Autodesk Inventor part; units mm, degrees
(part 2 of 3)
  line L370 (-43.7992, -26.7716) -> (-40.2132, -24.3987)
  spline S220 degree 2 poles (-43.3093, -22.1277) (-42.5945, -21.7354) (-41.4383, -21.9952) (-41.1231, -22.5695) knots 0 0 0 1 2 2 2
  spline S221 degree 2 poles (-41.1231, -22.5695) (-40.7995, -23.159) (-41.2324, -24.2751) (-41.9227, -24.654) knots 0 0 0 1 2 2 2
  spline S222 degree 2 poles (-41.9227, -24.654) (-42.6314, -25.043) (-43.7988, -24.7774) (-44.1106, -24.2092) knots 0 0 0 1 2 2 2
  spline S223 degree 2 poles (-44.1106, -24.2092) (-44.4258, -23.6349) (-44.0211, -22.5184) (-43.3093, -22.1277) knots 0 0 0 1 2 2 2
  spline S224 degree 2 poles (-43.0394, -22.6196) (-43.5892, -22.9214) (-43.9042, -23.6149) (-43.7013, -23.9846) knots 0 0 0 1 2 2 2
  spline S225 degree 2 poles (-43.7013, -23.9846) (-43.4984, -24.3542) (-42.7425, -24.464) (-42.1927, -24.1622) knots 0 0 0 1 2 2 2
  spline S226 degree 2 poles (-42.1927, -24.1622) (-41.6581, -23.8688) (-41.3296, -23.1638) (-41.5325, -22.7941) knots 0 0 0 1 2 2 2
  spline S227 degree 2 poles (-41.5325, -22.7941) (-41.7337, -22.4276) (-42.4957, -22.3211) (-43.0394, -22.6196) knots 0 0 0 1 2 2 2
  line L371 (-45.2535, -20.4403) -> (-45.2415, -20.4655)
  spline S228 degree 2 poles (-45.2415, -20.4655) (-45.2302, -20.5296) (-45.178, -20.6552) (-45.1375, -20.7401) knots 0 0 0 1 2 2 2
  spline S229 degree 2 poles (-45.1375, -20.7401) (-45.0429, -20.9383) (-44.6839, -21.2457) (-44.4301, -21.3408) knots 0 0 0 1 2 2 2
  line L372 (-44.4301, -21.3408) -> (-42.3638, -20.355)
  line L373 (-42.3638, -20.355) -> (-42.1297, -20.8456)
  line L374 (-42.1297, -20.8456) -> (-45.042, -22.2351)
  line L375 (-45.042, -22.2351) -> (-45.2761, -21.7445)
  line L376 (-45.2761, -21.7445) -> (-44.842, -21.5374)
  spline S230 degree 2 poles (-44.842, -21.5374) (-45.2086, -21.3841) (-45.5942, -21.0777) (-45.6842, -20.889) knots 0 0 0 1 2 2 2
  spline S231 degree 2 poles (-45.6842, -20.889) (-45.7202, -20.8135) (-45.7499, -20.7351) (-45.763, -20.6834) knots 0 0 0 1 2 2 2
  line L377 (-45.763, -20.6834) -> (-45.2535, -20.4403)
  spline S232 degree 2 poles (-45.6388, -17.058) (-44.8904, -16.7524) (-43.7153, -17.1043) (-43.4927, -17.6495) knots 0 0 0 1 2 2 2
  spline S233 degree 2 poles (-43.4927, -17.6495) (-43.4018, -17.8721) (-43.3654, -18.2562) (-43.3994, -18.4771) knots 0 0 0 1 2 2 2
  line L378 (-43.3994, -18.4771) -> (-42.1477, -17.9659)
  line L379 (-42.1477, -17.9659) -> (-41.9422, -18.4692)
  line L380 (-41.9422, -18.4692) -> (-46.0294, -20.1384)
  line L381 (-46.0294, -20.1384) -> (-46.235, -19.6351)
  line L382 (-46.235, -19.6351) -> (-45.9221, -19.5074)
  spline S234 degree 2 poles (-45.9221, -19.5074) (-46.1694, -19.3901) (-46.5823, -19.0242) (-46.6917, -18.7565) knots 0 0 0 1 2 2 2
  spline S235 degree 2 poles (-46.6917, -18.7565) (-46.9012, -18.2435) (-46.3227, -17.3373) (-45.6388, -17.058) knots 0 0 0 1 2 2 2
  spline S236 degree 2 poles (-45.3687, -17.5537) (-45.8816, -17.7631) (-46.3131, -18.3195) (-46.1642, -18.6841) knots 0 0 0 1 2 2 2
  spline S237 degree 2 poles (-46.1642, -18.6841) (-46.0772, -18.897) (-45.7235, -19.2193) (-45.5027, -19.3361) knots 0 0 0 1 2 2 2
  line L383 (-45.5027, -19.3361) -> (-43.8058, -18.6431)
  spline S238 degree 2 poles (-43.8058, -18.6431) (-43.7926, -18.4081) (-43.8363, -18.0985) (-43.9101, -17.9178) knots 0 0 0 1 2 2 2
  spline S239 degree 2 poles (-43.9101, -17.9178) (-44.0695, -17.5275) (-44.8202, -17.3297) (-45.3687, -17.5537) knots 0 0 0 1 2 2 2
  line L384 (-45.0446, -13.4768) -> (-44.8746, -13.9931)
  line L385 (-44.8746, -13.9931) -> (-46.6223, -14.5683)
  spline S240 degree 2 poles (-46.6223, -14.5683) (-46.8341, -14.638) (-47.1852, -14.7975) (-47.2748, -14.893) knots 0 0 0 1 2 2 2
  spline S241 degree 2 poles (-47.2748, -14.893) (-47.3699, -14.994) (-47.4084, -15.2562) (-47.3452, -15.4481) knots 0 0 0 1 2 2 2
  spline S242 degree 2 poles (-47.3452, -15.4481) (-47.2821, -15.6401) (-46.9429, -15.9797) (-46.7131, -16.1205) knots 0 0 0 1 2 2 2
  line L386 (-46.7131, -16.1205) -> (-44.4226, -15.3668)
  line L387 (-44.4226, -15.3668) -> (-44.2527, -15.8831)
  line L388 (-44.2527, -15.8831) -> (-48.5192, -17.2872)
  line L389 (-48.5192, -17.2872) -> (-48.6892, -16.7708)
  line L390 (-48.6892, -16.7708) -> (-47.1467, -16.2632)
  spline S243 degree 2 poles (-47.1467, -16.2632) (-47.4315, -16.1002) (-47.797, -15.7252) (-47.8798, -15.4736) knots 0 0 0 1 2 2 2
  spline S244 degree 2 poles (-47.8798, -15.4736) (-48.0279, -15.0235) (-47.5999, -14.3177) (-47.0339, -14.1314) knots 0 0 0 1 2 2 2
  line L391 (-47.0339, -14.1314) -> (-45.0446, -13.4768)
  spline S245 degree 2 poles (-47.472, -10.5709) (-46.6817, -10.3701) (-45.6275, -10.9113) (-45.4662, -11.5462) knots 0 0 0 1 2 2 2
  spline S246 degree 2 poles (-45.4662, -11.5462) (-45.3006, -12.1981) (-45.9993, -13.1701) (-46.7626, -13.3639) knots 0 0 0 1 2 2 2
  spline S247 degree 2 poles (-46.7626, -13.3639) (-47.5462, -13.563) (-48.6097, -13.0134) (-48.7693, -12.3852) knots 0 0 0 1 2 2 2
  spline S248 degree 2 poles (-48.7693, -12.3852) (-48.9305, -11.7502) (-48.2589, -10.7707) (-47.472, -10.5709) knots 0 0 0 1 2 2 2
  spline S249 degree 2 poles (-47.3339, -11.1146) (-47.9418, -11.269) (-48.4205, -11.8616) (-48.3167, -12.2702) knots 0 0 0 1 2 2 2
  spline S250 degree 2 poles (-48.3167, -12.2702) (-48.2129, -12.6789) (-47.5086, -12.9746) (-46.9007, -12.8202) knots 0 0 0 1 2 2 2
  spline S251 degree 2 poles (-46.9007, -12.8202) (-46.3097, -12.6701) (-45.815, -12.0698) (-45.9188, -11.6612) knots 0 0 0 1 2 2 2
  spline S252 degree 2 poles (-45.9188, -11.6612) (-46.0217, -11.2559) (-46.7327, -10.9619) (-47.3339, -11.1146) knots 0 0 0 1 2 2 2
  spline S253 degree 2 poles (-49.7235, -5.5011) (-49.4475, -5.4621) (-48.9228, -5.5884) (-48.7254, -5.7399) knots 0 0 0 1 2 2 2
  spline S254 degree 2 poles (-48.7254, -5.7399) (-48.4768, -5.93) (-48.168, -6.4951) (-48.1036, -6.9505) knots 0 0 0 1 2 2 2
  line L392 (-48.1036, -6.9505) -> (-48.0357, -7.4301)
  line L393 (-48.0357, -7.4301) -> (-46.4486, -7.2054)
  line L394 (-46.4486, -7.2054) -> (-46.3685, -7.7713)
  line L395 (-46.3685, -7.7713) -> (-50.626, -8.374)
  line L396 (-50.626, -8.374) -> (-50.7774, -7.3044)
  spline S255 degree 2 poles (-50.7774, -7.3044) (-50.8312, -6.9249) (-50.7822, -6.376) (-50.6695, -6.1524) knots 0 0 0 1 2 2 2
  spline S256 degree 2 poles (-50.6695, -6.1524) (-50.5411, -5.8914) (-50.0789, -5.5515) (-49.7235, -5.5011) knots 0 0 0 1 2 2 2
  spline S257 degree 2 poles (-49.6228, -6.0887) (-49.8436, -6.1199) (-50.1464, -6.3177) (-50.2279, -6.4876) knots 0 0 0 1 2 2 2
  spline S258 degree 2 poles (-50.2279, -6.4876) (-50.2986, -6.6348) (-50.3202, -7.0039) (-50.2826, -7.2696) knots 0 0 0 1 2 2 2
  line L397 (-50.2826, -7.2696) -> (-50.2162, -7.7388)
  line L398 (-50.2162, -7.7388) -> (-48.5187, -7.4985)
  line L399 (-48.5187, -7.4985) -> (-48.5734, -7.1121)
  spline S259 degree 2 poles (-48.5734, -7.1121) (-48.6222, -6.7671) (-48.7927, -6.3583) (-48.9572, -6.2408) knots 0 0 0 1 2 2 2
  spline S260 degree 2 poles (-48.9572, -6.2408) (-49.1029, -6.1312) (-49.4192, -6.0599) (-49.6228, -6.0887) knots 0 0 0 1 2 2 2
  line L400 (-46.9725, -2.0535) -> (-46.934, -2.5957)
  line L401 (-46.934, -2.5957) -> (-48.7693, -2.7261)
  spline S261 degree 2 poles (-48.7693, -2.7261) (-48.9917, -2.7419) (-49.3711, -2.8107) (-49.4814, -2.8814) knots 0 0 0 1 2 2 2
  spline S262 degree 2 poles (-49.4814, -2.8814) (-49.5983, -2.9561) (-49.6997, -3.2009) (-49.6854, -3.4025) knots 0 0 0 1 2 2 2
  spline S263 degree 2 poles (-49.6854, -3.4025) (-49.6711, -3.6041) (-49.4252, -4.0163) (-49.2369, -4.209) knots 0 0 0 1 2 2 2
  line L402 (-49.2369, -4.209) -> (-46.8316, -4.0382)
  line L403 (-46.8316, -4.0382) -> (-46.7931, -4.5805)
  line L404 (-46.7931, -4.5805) -> (-51.2735, -4.8986)
  line L405 (-51.2735, -4.8986) -> (-51.312, -4.3564)
  line L406 (-51.312, -4.3564) -> (-49.6922, -4.2414)
  spline S264 degree 2 poles (-49.6922, -4.2414) (-49.9285, -4.0136) (-50.1912, -3.5607) (-50.21, -3.2965) knots 0 0 0 1 2 2 2
  spline S265 degree 2 poles (-50.21, -3.2965) (-50.2435, -2.8238) (-49.6559, -2.2441) (-49.0615, -2.2019) knots 0 0 0 1 2 2 2
  line L407 (-49.0615, -2.2019) -> (-46.9725, -2.0535)
  line L408 (-50.2328, 1.2276) -> (-45.81, -0.4878)
  line L409 (-45.81, -0.4878) -> (-45.8074, -1.0697)
  line L410 (-45.8074, -1.0697) -> (-47.155, -0.4973)
  line L411 (-47.155, -0.4973) -> (-50.2196, -1.682)
  line L412 (-50.2196, -1.682) -> (-50.2223, -1.0966)
  line L413 (-50.2223, -1.0966) -> (-47.8359, -0.2042)
  line L414 (-47.8359, -0.2042) -> (-50.2303, 0.6631)
  line L415 (-50.2303, 0.6631) -> (-50.2328, 1.2276)
  spline S266 degree 2 poles (-46.8557, 2.5183) (-46.8735, 2.1947) (-47.0782, 1.6441) (-47.1858, 1.465) knots 0 0 0 1 2 2 2
  line L416 (-47.1858, 1.465) -> (-47.7947, 1.4984)
  line L417 (-47.7947, 1.4984) -> (-47.7931, 1.5263)
  spline S267 degree 2 poles (-47.7931, 1.5263) (-47.7336, 1.5928) (-47.5911, 1.7734) (-47.5095, 1.926) knots 0 0 0 1 2 2 2
  spline S268 degree 2 poles (-47.5095, 1.926) (-47.4359, 2.0581) (-47.3201, 2.3867) (-47.3104, 2.5642) knots 0 0 0 1 2 2 2
  spline S269 degree 2 poles (-47.3104, 2.5642) (-47.3033, 2.6929) (-47.3462, 2.9919) (-47.3911, 3.0642) knots 0 0 0 1 2 2 2
  spline S270 degree 2 poles (-47.3911, 3.0642) (-47.4517, 3.1687) (-47.5963, 3.2674) (-47.7494, 3.2758) knots 0 0 0 1 2 2 2
  spline S271 degree 2 poles (-47.7494, 3.2758) (-47.9408, 3.2863) (-48.1506, 3.0884) (-48.2314, 2.8241) knots 0 0 0 1 2 2 2
  spline S272 degree 2 poles (-48.2314, 2.8241) (-48.2615, 2.7211) (-48.3494, 2.3909) (-48.3955, 2.2503) knots 0 0 0 1 2 2 2
  spline S273 degree 2 poles (-48.3955, 2.2503) (-48.5236, 1.8874) (-48.9873, 1.5779) (-49.3039, 1.5953) knots 0 0 0 1 2 2 2
  spline S274 degree 2 poles (-49.3039, 1.5953) (-49.7423, 1.6193) (-50.2525, 2.3069) (-50.2227, 2.8497) knots 0 0 0 1 2 2 2
  spline S275 degree 2 poles (-50.2227, 2.8497) (-50.208, 3.1176) (-50.046, 3.6531) (-49.935, 3.832) knots 0 0 0 1 2 2 2
  line L418 (-49.935, 3.832) -> (-49.3539, 3.8001)
  line L419 (-49.3539, 3.8001) -> (-49.3554, 3.7723)
  spline S276 degree 2 poles (-49.3554, 3.7723) (-49.5339, 3.5727) (-49.7532, 3.0752) (-49.7675, 2.8142) knots 0 0 0 1 2 2 2
  spline S277 degree 2 poles (-49.7675, 2.8142) (-49.7822, 2.5463) (-49.5763, 2.1651) (-49.3501, 2.1527) knots 0 0 0 1 2 2 2
  spline S278 degree 2 poles (-49.3501, 2.1527) (-49.1448, 2.1414) (-48.9345, 2.3497) (-48.8585, 2.5898) knots 0 0 0 1 2 2 2
  spline S279 degree 2 poles (-48.8585, 2.5898) (-48.8207, 2.7064) (-48.7416, 3.0022) (-48.6944, 3.1636) knots 0 0 0 1 2 2 2
  spline S280 degree 2 poles (-48.6944, 3.1636) (-48.5844, 3.5136) (-48.1505, 3.8527) (-47.7921, 3.833) knots 0 0 0 1 2 2 2
  spline S281 degree 2 poles (-47.7921, 3.833) (-47.5834, 3.8216) (-47.2235, 3.6378) (-47.0966, 3.4703) knots 0 0 0 1 2 2 2
  spline S282 degree 2 poles (-47.0966, 3.4703) (-46.9633, 3.292) (-46.8376, 2.8488) (-46.8557, 2.5183) knots 0 0 0 1 2 2 2
  line L420 (-46.7514, 4.8356) -> (-46.8042, 4.2945)
  line L421 (-46.8042, 4.2945) -> (-50.0157, 4.6079)
  line L422 (-50.0157, 4.6079) -> (-49.9629, 5.149)
  line L423 (-49.9629, 5.149) -> (-46.7514, 4.8356)
  line L424 (-50.4932, 5.2392) -> (-50.5531, 4.6254)
  line L425 (-50.5531, 4.6254) -> (-51.115, 4.6802)
  line L426 (-51.115, 4.6802) -> (-51.0551, 5.2941)
  line L427 (-51.0551, 5.2941) -> (-50.4932, 5.2392)
  spline S283 degree 2 poles (-46.4195, 6.8888) (-46.4664, 6.5576) (-46.7476, 6.0378) (-46.9825, 5.8705) knots 0 0 0 1 2 2 2
  spline S284 degree 2 poles (-46.9825, 5.8705) (-47.2139, 5.7027) (-47.8726, 5.5742) (-48.2935, 5.6338) knots 0 0 0 1 2 2 2
  spline S285 degree 2 poles (-48.2935, 5.6338) (-48.7145, 5.6934) (-49.2968, 6.0047) (-49.477, 6.2237) knots 0 0 0 1 2 2 2
  spline S286 degree 2 poles (-49.477, 6.2237) (-49.6606, 6.4433) (-49.8052, 7.0374) (-49.7593, 7.3618) knots 0 0 0 1 2 2 2
  spline S287 degree 2 poles (-49.7593, 7.3618) (-49.7221, 7.624) (-49.5044, 8.0929) (-49.3809, 8.269) knots 0 0 0 1 2 2 2
  line L428 (-49.3809, 8.269) -> (-48.7771, 8.1835)
  line L429 (-48.7771, 8.1835) -> (-48.7815, 8.1524)
  spline S288 degree 2 poles (-48.7815, 8.1524) (-48.8381, 8.1006) (-48.9877, 7.9388) (-49.0714, 7.8204) knots 0 0 0 1 2 2 2
  spline S289 degree 2 poles (-49.0714, 7.8204) (-49.1427, 7.7144) (-49.272, 7.423) (-49.2915, 7.285) knots 0 0 0 1 2 2 2
  spline S290 degree 2 poles (-49.2915, 7.285) (-49.3506, 6.8675) (-48.7911, 6.2709) (-48.2149, 6.1893) knots 0 0 0 1 2 2 2
  spline S291 degree 2 poles (-48.2149, 6.1893) (-47.6525, 6.1097) (-46.9517, 6.5102) (-46.8902, 6.9449) knots 0 0 0 1 2 2 2
  spline S292 degree 2 poles (-46.8902, 6.9449) (-46.853, 7.2071) (-47.003, 7.714) (-47.1461, 7.9208) knots 0 0 0 1 2 2 2
  line L430 (-47.1461, 7.9208) -> (-47.1417, 7.9519)
  line L431 (-47.1417, 7.9519) -> (-46.538, 7.8664)
  spline S293 degree 2 poles (-46.538, 7.8664) (-46.5112, 7.7816) (-46.4385, 7.525) (-46.428, 7.4249) knots 0 0 0 1 2 2 2
  spline S294 degree 2 poles (-46.428, 7.4249) (-46.4062, 7.2811) (-46.3955, 7.0579) (-46.4195, 6.8888) knots 0 0 0 1 2 2 2
  spline S295 degree 2 poles (-46.0194, 9.166) (-46.0831, 8.8482) (-46.3641, 8.3324) (-46.4961, 8.1705) knots 0 0 0 1 2 2 2
  line L432 (-46.4961, 8.1705) -> (-47.094, 8.2903)
  line L433 (-47.094, 8.2903) -> (-47.0885, 8.3176)
  spline S296 degree 2 poles (-47.0885, 8.3176) (-47.0202, 8.375) (-46.8534, 8.5335) (-46.7508, 8.6728) knots 0 0 0 1 2 2 2
  spline S297 degree 2 poles (-46.7508, 8.6728) (-46.6592, 8.7931) (-46.4978, 9.1019) (-46.4629, 9.2762) knots 0 0 0 1 2 2 2
  spline S298 degree 2 poles (-46.4629, 9.2762) (-46.4376, 9.4026) (-46.4375, 9.7046) (-46.4716, 9.7826) knots 0 0 0 1 2 2 2
  spline S299 degree 2 poles (-46.4716, 9.7826) (-46.5167, 9.8947) (-46.6458, 10.0129) (-46.7961, 10.0431) knots 0 0 0 1 2 2 2
  spline S300 degree 2 poles (-46.7961, 10.0431) (-46.984, 10.0807) (-47.2199, 9.9147) (-47.3375, 9.6646) knots 0 0 0 1 2 2 2
  spline S301 degree 2 poles (-47.3375, 9.6646) (-47.382, 9.5669) (-47.516, 9.2526) (-47.5817, 9.1201) knots 0 0 0 1 2 2 2
  spline S302 degree 2 poles (-47.5817, 9.1201) (-47.7601, 8.7791) (-48.2632, 8.5388) (-48.5741, 8.6011) knots 0 0 0 1 2 2 2
  spline S303 degree 2 poles (-48.5741, 8.6011) (-49.0046, 8.6873) (-49.4117, 9.4406) (-49.3049, 9.9736) knots 0 0 0 1 2 2 2
  spline S304 degree 2 poles (-49.3049, 9.9736) (-49.2521, 10.2366) (-49.0155, 10.7436) (-48.8801, 10.9049) knots 0 0 0 1 2 2 2
  line L434 (-48.8801, 10.9049) -> (-48.3096, 10.7905)
  line L435 (-48.3096, 10.7905) -> (-48.315, 10.7632)
  spline S305 degree 2 poles (-48.315, 10.7632) (-48.5201, 10.5911) (-48.808, 10.1299) (-48.8593, 9.8736) knots 0 0 0 1 2 2 2
  spline S306 degree 2 poles (-48.8593, 9.8736) (-48.912, 9.6105) (-48.7625, 9.2039) (-48.5404, 9.1594) knots 0 0 0 1 2 2 2
  spline S307 degree 2 poles (-48.5404, 9.1594) (-48.3389, 9.119) (-48.101, 9.2952) (-47.9916, 9.5221) knots 0 0 0 1 2 2 2
  spline S308 degree 2 poles (-47.9916, 9.5221) (-47.9375, 9.6321) (-47.8171, 9.9136) (-47.7474, 10.0666) knots 0 0 0 1 2 2 2
  spline S309 degree 2 poles (-47.7474, 10.0666) (-47.5887, 10.3973) (-47.1109, 10.6712) (-46.759, 10.6007) knots 0 0 0 1 2 2 2
  spline S310 degree 2 poles (-46.759, 10.6007) (-46.554, 10.5596) (-46.224, 10.3265) (-46.1223, 10.1426) knots 0 0 0 1 2 2 2
  spline S311 degree 2 poles (-46.1223, 10.1426) (-46.0157, 9.9471) (-45.9544, 9.4906) (-46.0194, 9.166) knots 0 0 0 1 2 2 2
  line L436 (-45.1171, 18.2845) -> (-45.6167, 16.9164)
  line L437 (-45.6167, 16.9164) -> (-44.2485, 16.4167)
  line L438 (-44.2485, 16.4167) -> (-44.4135, 15.965)
  line L439 (-44.4135, 15.965) -> (-45.7817, 16.4647)
  line L440 (-45.7817, 16.4647) -> (-46.2813, 15.0965)
  line L441 (-46.2813, 15.0965) -> (-46.7166, 15.2554)
  line L442 (-46.7166, 15.2554) -> (-46.217, 16.6236)
  line L443 (-46.217, 16.6236) -> (-47.5852, 17.1233)
  line L444 (-47.5852, 17.1233) -> (-47.4202, 17.575)
  line L445 (-47.4202, 17.575) -> (-46.052, 17.0753)
  line L446 (-46.052, 17.0753) -> (-45.5524, 18.4435)
  line L447 (-45.5524, 18.4435) -> (-45.1171, 18.2845)
  line L448 (-43.2576, 22.3305) -> (-43.8802, 21.0137)
  line L449 (-43.8802, 21.0137) -> (-42.5634, 20.3911)
  line L450 (-42.5634, 20.3911) -> (-42.7689, 19.9564)
  line L451 (-42.7689, 19.9564) -> (-44.0857, 20.5789)
  line L452 (-44.0857, 20.5789) -> (-44.7083, 19.2621)
  line L453 (-44.7083, 19.2621) -> (-45.1273, 19.4602)
  line L454 (-45.1273, 19.4602) -> (-44.5047, 20.777)
  line L455 (-44.5047, 20.777) -> (-45.8215, 21.3996)
  line L456 (-45.8215, 21.3996) -> (-45.616, 21.8343)
  line L457 (-45.616, 21.8343) -> (-44.2992, 21.2118)
  line L458 (-44.2992, 21.2118) -> (-43.6766, 22.5286)
  line L459 (-43.6766, 22.5286) -> (-43.2576, 22.3305)
  line L460 (-41.0363, 26.1896) -> (-41.7766, 24.9352)
  line L461 (-41.7766, 24.9352) -> (-40.5222, 24.1949)
  line L462 (-40.5222, 24.1949) -> (-40.7666, 23.7808)
  line L463 (-40.7666, 23.7808) -> (-42.021, 24.5211)
  line L464 (-42.021, 24.5211) -> (-42.7613, 23.2666)
  line L465 (-42.7613, 23.2666) -> (-43.1604, 23.5022)
  line L466 (-43.1604, 23.5022) -> (-42.4201, 24.7566)
  line L467 (-42.4201, 24.7566) -> (-43.6745, 25.4969)
  line L468 (-43.6745, 25.4969) -> (-43.4301, 25.911)
  line L469 (-43.4301, 25.911) -> (-42.1757, 25.1707)
  line L470 (-42.1757, 25.1707) -> (-41.4354, 26.4252)
  line L471 (-41.4354, 26.4252) -> (-41.0363, 26.1896)
  spline S312 degree 2 poles (-37.5248, 33.0844) (-37.3102, 32.9065) (-37.0507, 32.4334) (-37.03, 32.1853) knots 0 0 0 1 2 2 2
  spline S313 degree 2 poles (-37.03, 32.1853) (-37.0033, 31.8735) (-37.2136, 31.2649) (-37.5072, 30.9108) knots 0 0 0 1 2 2 2
  line L472 (-37.5072, 30.9108) -> (-37.8163, 30.5379)
  line L473 (-37.8163, 30.5379) -> (-36.5822, 29.5149)
  line L474 (-36.5822, 29.5149) -> (-36.9469, 29.0749)
  line L475 (-36.9469, 29.0749) -> (-40.2574, 31.8192)
  line L476 (-40.2574, 31.8192) -> (-39.568, 32.6508)
  spline S314 degree 2 poles (-39.568, 32.6508) (-39.3234, 32.9459) (-38.8843, 33.279) (-38.6431, 33.3461) knots 0 0 0 1 2 2 2
  spline S315 degree 2 poles (-38.6431, 33.3461) (-38.3636, 33.4267) (-37.8012, 33.3135) (-37.5248, 33.0844) knots 0 0 0 1 2 2 2
  spline S316 degree 2 poles (-37.8917, 32.6145) (-38.0634, 32.7569) (-38.4134, 32.8479) (-38.594, 32.7939) knots 0 0 0 1 2 2 2
  spline S317 degree 2 poles (-38.594, 32.7939) (-38.7505, 32.7471) (-39.0381, 32.5148) (-39.2093, 32.3082) knots 0 0 0 1 2 2 2
  line L477 (-39.2093, 32.3082) -> (-39.5118, 31.9433)
  line L478 (-39.5118, 31.9433) -> (-38.1919, 30.8492)
  line L479 (-38.1919, 30.8492) -> (-37.9428, 31.1497)
  spline S318 degree 2 poles (-37.9428, 31.1497) (-37.7204, 31.4179) (-37.5327, 31.8191) (-37.5564, 32.0198) knots 0 0 0 1 2 2 2
  spline S319 degree 2 poles (-37.5564, 32.0198) (-37.5734, 32.2013) (-37.7334, 32.4833) (-37.8917, 32.6145) knots 0 0 0 1 2 2 2
  spline S320 degree 2 poles (-33.8792, 33.073) (-33.8895, 32.9914) (-33.9168, 32.7097) (-33.9509, 32.5979) knots 0 0 0 1 2 2 2
  spline S321 degree 2 poles (-33.9509, 32.5979) (-33.9937, 32.4416) (-34.1204, 32.1918) (-34.2885, 32.015) knots 0 0 0 1 2 2 2
  spline S322 degree 2 poles (-34.2885, 32.015) (-34.4253, 31.871) (-34.7811, 31.714) (-34.9733, 31.7091) knots 0 0 0 1 2 2 2
  spline S323 degree 2 poles (-34.9733, 31.7091) (-35.1581, 31.7069) (-35.549, 31.862) (-35.7056, 32.0108) knots 0 0 0 1 2 2 2
  spline S324 degree 2 poles (-35.7056, 32.0108) (-35.9481, 32.2413) (-36.0972, 32.7723) (-35.9845, 33.0882) knots 0 0 0 1 2 2 2
  spline S325 degree 2 poles (-35.9845, 33.0882) (-35.8883, 33.3717) (-35.4476, 33.972) (-35.1701, 34.2995) knots 0 0 0 1 2 2 2
  line L480 (-35.1701, 34.2995) -> (-35.2459, 34.3715)
  spline S326 degree 2 poles (-35.2459, 34.3715) (-35.3823, 34.5011) (-35.6307, 34.5786) (-35.7507, 34.5484) knots 0 0 0 1 2 2 2
  spline S327 degree 2 poles (-35.7507, 34.5484) (-35.8707, 34.5182) (-36.1075, 34.3298) (-36.2179, 34.2136) knots 0 0 0 1 2 2 2
  spline S328 degree 2 poles (-36.2179, 34.2136) (-36.3475, 34.0772) (-36.6171, 33.6316) (-36.714, 33.3728) knots 0 0 0 1 2 2 2
  line L481 (-36.714, 33.3728) -> (-36.7356, 33.35)
  line L482 (-36.7356, 33.35) -> (-37.1373, 33.7317)
  spline S329 degree 2 poles (-37.1373, 33.7317) (-37.0644, 33.8691) (-36.7537, 34.3478) (-36.5641, 34.5474) knots 0 0 0 1 2 2 2
  spline S330 degree 2 poles (-36.5641, 34.5474) (-36.3337, 34.7899) (-35.9434, 35.0488) (-35.7201, 35.0865) knots 0 0 0 1 2 2 2
  spline S331 degree 2 poles (-35.7201, 35.0865) (-35.5017, 35.1242) (-35.076, 34.96) (-34.8563, 34.7512) knots 0 0 0 1 2 2 2
  line L483 (-34.8563, 34.7512) -> (-33.2572, 33.2319)
  line L484 (-33.2572, 33.2319) -> (-33.6317, 32.8378)
  line L485 (-33.6317, 32.8378) -> (-33.8792, 33.073)
  line L486 (-34.2076, 33.385) -> (-34.8568, 34.0019)
  spline S332 degree 2 poles (-34.8568, 34.0019) (-34.9786, 33.8484) (-35.3413, 33.3807) (-35.4281, 33.2084) knots 0 0 0 1 2 2 2
  spline S333 degree 2 poles (-35.4281, 33.2084) (-35.5289, 33.0062) (-35.5238, 32.612) (-35.347, 32.444) knots 0 0 0 1 2 2 2
  spline S334 degree 2 poles (-35.347, 32.444) (-35.1449, 32.2519) (-34.7242, 32.2849) (-34.5178, 32.5021) knots 0 0 0 1 2 2 2
  spline S335 degree 2 poles (-34.5178, 32.5021) (-34.3426, 32.6865) (-34.2137, 33.1409) (-34.2076, 33.385) knots 0 0 0 1 2 2 2
  line L487 (-33.2738, 36.8584) -> (-33.2941, 36.8393)
  spline S336 degree 2 poles (-33.2941, 36.8393) (-33.3517, 36.809) (-33.4554, 36.7209) (-33.5239, 36.6564) knots 0 0 0 1 2 2 2
  spline S337 degree 2 poles (-33.5239, 36.6564) (-33.6838, 36.5059) (-33.867, 36.0702) (-33.8801, 35.7994) knots 0 0 0 1 2 2 2
  line L488 (-33.8801, 35.7994) -> (-32.3108, 34.1325)
  line L489 (-32.3108, 34.1325) -> (-32.7066, 33.7599)
  line L490 (-32.7066, 33.7599) -> (-34.9184, 36.1093)
  line L491 (-34.9184, 36.1093) -> (-34.5226, 36.4819)
  line L492 (-34.5226, 36.4819) -> (-34.193, 36.1318)
  spline S338 degree 2 poles (-34.193, 36.1318) (-34.1589, 36.5276) (-33.9848, 36.9883) (-33.8325, 37.1316) knots 0 0 0 1 2 2 2
  spline S339 degree 2 poles (-33.8325, 37.1316) (-33.7716, 37.1889) (-33.706, 37.2412) (-33.6607, 37.2694) knots 0 0 0 1 2 2 2
  line L493 (-33.6607, 37.2694) -> (-33.2738, 36.8584)
  line L494 (-30.722, 35.5701) -> (-31.1314, 35.2124)
  line L495 (-31.1314, 35.2124) -> (-33.2546, 37.6421)
  line L496 (-33.2546, 37.6421) -> (-32.8453, 37.9998)
  line L497 (-32.8453, 37.9998) -> (-30.722, 35.5701)
  line L498 (-33.1695, 38.4292) -> (-33.6339, 38.0233)
  line L499 (-33.6339, 38.0233) -> (-34.0054, 38.4484)
  line L500 (-34.0054, 38.4484) -> (-33.541, 38.8542)
  line L501 (-33.541, 38.8542) -> (-33.1695, 38.4292)
  spline S340 degree 2 poles (-29.3916, 36.5778) (-29.6444, 36.3751) (-30.1911, 36.1602) (-30.3963, 36.1208) knots 0 0 0 1 2 2 2
  line L502 (-30.3963, 36.1208) -> (-30.7777, 36.5966)
  line L503 (-30.7777, 36.5966) -> (-30.7559, 36.614)
  spline S341 degree 2 poles (-30.7559, 36.614) (-30.6667, 36.6141) (-30.4371, 36.6285) (-30.2689, 36.6695) knots 0 0 0 1 2 2 2
  spline S342 degree 2 poles (-30.2689, 36.6695) (-30.1215, 36.7028) (-29.7995, 36.8359) (-29.6608, 36.9471) knots 0 0 0 1 2 2 2
  spline S343 degree 2 poles (-29.6608, 36.9471) (-29.5602, 37.0277) (-29.3661, 37.2592) (-29.3423, 37.3408) knots 0 0 0 1 2 2 2
  spline S344 degree 2 poles (-29.3423, 37.3408) (-29.3048, 37.4557) (-29.3279, 37.6293) (-29.4238, 37.7489) knots 0 0 0 1 2 2 2
  spline S345 degree 2 poles (-29.4238, 37.7489) (-29.5437, 37.8985) (-29.831, 37.9227) (-30.0818, 37.8065) knots 0 0 0 1 2 2 2
  spline S346 degree 2 poles (-30.0818, 37.8065) (-30.1786, 37.7601) (-30.4832, 37.6053) (-30.6186, 37.5458) knots 0 0 0 1 2 2 2
  spline S347 degree 2 poles (-30.6186, 37.5458) (-30.9744, 37.3991) (-31.5144, 37.5379) (-31.7127, 37.7853) knots 0 0 0 1 2 2 2
  spline S348 degree 2 poles (-31.7127, 37.7853) (-31.9874, 38.1278) (-31.8157, 38.9666) (-31.3915, 39.3066) knots 0 0 0 1 2 2 2
  spline S349 degree 2 poles (-31.3915, 39.3066) (-31.1822, 39.4745) (-30.6752, 39.7112) (-30.4679, 39.7478) knots 0 0 0 1 2 2 2
  line L504 (-30.4679, 39.7478) -> (-30.1039, 39.2938)
  line L505 (-30.1039, 39.2938) -> (-30.1257, 39.2763)
  spline S350 degree 2 poles (-30.1257, 39.2763) (-30.3934, 39.2761) (-30.9103, 39.1074) (-31.1142, 38.9439) knots 0 0 0 1 2 2 2
  spline S351 degree 2 poles (-31.1142, 38.9439) (-31.3235, 38.7761) (-31.4701, 38.3684) (-31.3284, 38.1916) knots 0 0 0 1 2 2 2
  spline S352 degree 2 poles (-31.3284, 38.1916) (-31.1998, 38.0312) (-30.9043, 38.0136) (-30.6747, 38.1172) knots 0 0 0 1 2 2 2
  spline S353 degree 2 poles (-30.6747, 38.1172) (-30.5627, 38.1668) (-30.2896, 38.3053) (-30.1379, 38.3778) knots 0 0 0 1 2 2 2
  spline S354 degree 2 poles (-30.1379, 38.3778) (-29.8039, 38.5295) (-29.2617, 38.4326) (-29.0373, 38.1526) knots 0 0 0 1 2 2 2
  spline S355 degree 2 poles (-29.0373, 38.1526) (-28.9065, 37.9894) (-28.8032, 37.5988) (-28.8433, 37.3925) knots 0 0 0 1 2 2 2
  spline S356 degree 2 poles (-28.8433, 37.3925) (-28.8872, 37.1742) (-29.1333, 36.7849) (-29.3916, 36.5778) knots 0 0 0 1 2 2 2
  line L506 (-24.4232, 40.1825) -> (-26.5111, 38.8231)
  line L507 (-26.5111, 38.8231) -> (-28.8573, 42.4266)
  line L508 (-28.8573, 42.4266) -> (-28.3784, 42.7384)
  line L509 (-28.3784, 42.7384) -> (-26.3098, 39.5612)
  line L510 (-26.3098, 39.5612) -> (-24.7008, 40.6088)
  line L511 (-24.7008, 40.6088) -> (-24.4232, 40.1825)
  spline S357 degree 2 poles (-22.5484, 43.0918) (-22.1491, 42.3809) (-22.3976, 41.2222) (-22.9688, 40.9014) knots 0 0 0 1 2 2 2
  spline S358 degree 2 poles (-22.9688, 40.9014) (-23.5552, 40.5721) (-24.6754, 40.9941) (-25.061, 41.6807) knots 0 0 0 1 2 2 2
  spline S359 degree 2 poles (-25.061, 41.6807) (-25.4569, 42.3856) (-25.2027, 43.5555) (-24.6375, 43.8728) knots 0 0 0 1 2 2 2
  spline S360 degree 2 poles (-24.6375, 43.8728) (-24.0664, 44.1936) (-22.9459, 43.7998) (-22.5484, 43.0918) knots 0 0 0 1 2 2 2
  spline S361 degree 2 poles (-23.0375, 42.8171) (-23.3447, 43.364) (-24.0413, 43.6722) (-24.4089, 43.4657) knots 0 0 0 1 2 2 2
  spline S362 degree 2 poles (-24.4089, 43.4657) (-24.7765, 43.2593) (-24.879, 42.5023) (-24.5718, 41.9554) knots 0 0 0 1 2 2 2
  spline S363 degree 2 poles (-24.5718, 41.9554) (-24.2732, 41.4237) (-23.565, 41.1021) (-23.1974, 41.3086) knots 0 0 0 1 2 2 2
  spline S364 degree 2 poles (-23.1974, 41.3086) (-22.8328, 41.5133) (-22.7338, 42.2763) (-23.0375, 42.8171) knots 0 0 0 1 2 2 2
  line L512 (-19.0185, 42.9981) -> (-19.5097, 42.7652)
  line L513 (-19.5097, 42.7652) -> (-19.65, 43.0611)
  spline S365 degree 2 poles (-19.65, 43.0611) (-19.7186, 42.9129) (-19.8257, 42.7078) (-19.9137, 42.6006) knots 0 0 0 1 2 2 2
  spline S366 degree 2 poles (-19.9137, 42.6006) (-19.9937, 42.5009) (-20.1919, 42.3414) (-20.3398, 42.2712) knots 0 0 0 1 2 2 2
  spline S367 degree 2 poles (-20.3398, 42.2712) (-20.5791, 42.1577) (-21.0762, 42.1649) (-21.309, 42.2898) knots 0 0 0 1 2 2 2
  spline S368 degree 2 poles (-21.309, 42.2898) (-21.5417, 42.4147) (-21.9679, 42.9067) (-22.1426, 43.2751) knots 0 0 0 1 2 2 2
  spline S369 degree 2 poles (-22.1426, 43.2751) (-22.3248, 43.6592) (-22.3922, 44.3137) (-22.3191, 44.6068) knots 0 0 0 1 2 2 2
  spline S370 degree 2 poles (-22.3191, 44.6068) (-22.2481, 44.8719) (-21.9009, 45.3026) (-21.6521, 45.4206) knots 0 0 0 1 2 2 2
  spline S371 degree 2 poles (-21.6521, 45.4206) (-21.4349, 45.5236) (-21.0643, 45.5798) (-20.8371, 45.5642) knots 0 0 0 1 2 2 2
  line L514 (-20.8371, 45.5642) -> (-21.4343, 46.8236)
  line L515 (-21.4343, 46.8236) -> (-20.9432, 47.0565)
  line L516 (-20.9432, 47.0565) -> (-19.0185, 42.9981)
  line L517 (-19.8456, 43.4736) -> (-20.6445, 45.158)
  spline S372 degree 2 poles (-20.6445, 45.158) (-20.8689, 45.1596) (-21.1899, 45.0883) (-21.3568, 45.0092) knots 0 0 0 1 2 2 2
  spline S373 degree 2 poles (-21.3568, 45.0092) (-21.7346, 44.83) (-21.894, 44.0602) (-21.6402, 43.525) knots 0 0 0 1 2 2 2
  spline S374 degree 2 poles (-21.6402, 43.525) (-21.3953, 43.0086) (-20.8095, 42.6192) (-20.4475, 42.7909) knots 0 0 0 1 2 2 2
  spline S375 degree 2 poles (-20.4475, 42.7909) (-20.2554, 42.882) (-19.9486, 43.2435) (-19.8456, 43.4736) knots 0 0 0 1 2 2 2
  line L518 (-17.7002, 46.3939) -> (-17.726, 46.3834)
  spline S376 degree 2 poles (-17.726, 46.3834) (-17.7907, 46.3759) (-17.9192, 46.3313) (-18.0064, 46.2959) knots 0 0 0 1 2 2 2
  spline S377 degree 2 poles (-18.0064, 46.2959) (-18.2098, 46.2134) (-18.5382, 45.8734) (-18.6483, 45.6257) knots 0 0 0 1 2 2 2
  line L519 (-18.6483, 45.6257) -> (-17.7876, 43.5042)
  line L520 (-17.7876, 43.5042) -> (-18.2914, 43.2999)
  line L521 (-18.2914, 43.2999) -> (-19.5044, 46.2899)
  line L522 (-19.5044, 46.2899) -> (-19.0006, 46.4943)
  line L523 (-19.0006, 46.4943) -> (-18.8199, 46.0487)
  spline S378 degree 2 poles (-18.8199, 46.0487) (-18.645, 46.4054) (-18.3161, 46.772) (-18.1223, 46.8506) knots 0 0 0 1 2 2 2
  spline S379 degree 2 poles (-18.1223, 46.8506) (-18.0449, 46.882) (-17.9647, 46.907) (-17.9124, 46.917) knots 0 0 0 1 2 2 2
  line L524 (-17.9124, 46.917) -> (-17.7002, 46.3939)
  spline S380 degree 2 poles (-14.3235, 46.4777) (-14.0604, 45.7059) (-14.5158, 44.6118) (-15.1358, 44.4004) knots 0 0 0 1 2 2 2
  spline S381 degree 2 poles (-15.1358, 44.4004) (-15.7724, 44.1834) (-16.797, 44.8023) (-17.0511, 45.5477) knots 0 0 0 1 2 2 2
  spline S382 degree 2 poles (-17.0511, 45.5477) (-17.312, 46.3129) (-16.849, 47.4169) (-16.2355, 47.6261) knots 0 0 0 1 2 2 2
  spline S383 degree 2 poles (-16.2355, 47.6261) (-15.6155, 47.8375) (-14.5855, 47.2461) (-14.3235, 46.4777) knots 0 0 0 1 2 2 2
  spline S384 degree 2 poles (-14.8545, 46.2966) (-15.0569, 46.8903) (-15.6858, 47.3202) (-16.0849, 47.1841) knots 0 0 0 1 2 2 2
  spline S385 degree 2 poles (-16.0849, 47.1841) (-16.484, 47.048) (-16.7225, 46.3224) (-16.5201, 45.7288) knots 0 0 0 1 2 2 2
  spline S386 degree 2 poles (-16.5201, 45.7288) (-16.3233, 45.1516) (-15.6856, 44.7063) (-15.2865, 44.8424) knots 0 0 0 1 2 2 2
  spline S387 degree 2 poles (-15.2865, 44.8424) (-14.8907, 44.9773) (-14.6544, 45.7095) (-14.8545, 46.2966) knots 0 0 0 1 2 2 2
  line L525 (-10.8192, 45.7557) -> (-11.3446, 45.6162)
  line L526 (-11.3446, 45.6162) -> (-11.8165, 47.3946)
  spline S388 degree 2 poles (-11.8165, 47.3946) (-11.8737, 47.6101) (-12.0124, 47.9699) (-12.1026, 48.0649) knots 0 0 0 1 2 2 2
  spline S389 degree 2 poles (-12.1026, 48.0649) (-12.1978, 48.1658) (-12.4573, 48.2196) (-12.6526, 48.1677) knots 0 0 0 1 2 2 2
  spline S390 degree 2 poles (-12.6526, 48.1677) (-12.8479, 48.1159) (-13.2068, 47.7971) (-13.3608, 47.576) knots 0 0 0 1 2 2 2
  line L527 (-13.3608, 47.576) -> (-12.7423, 45.2453)
  line L528 (-12.7423, 45.2453) -> (-13.2677, 45.1059)
  line L529 (-13.2677, 45.1059) -> (-14.0954, 48.2247)
  line L530 (-14.0954, 48.2247) -> (-13.57, 48.3641)
  line L531 (-13.57, 48.3641) -> (-13.4779, 48.0172)
  spline S391 degree 2 poles (-13.4779, 48.0172) (-13.2985, 48.292) (-12.9028, 48.6349) (-12.6468, 48.7028) knots 0 0 0 1 2 2 2
  spline S392 degree 2 poles (-12.6468, 48.7028) (-12.1887, 48.8244) (-11.5092, 48.3558) (-11.3563, 47.7798) knots 0 0 0 1 2 2 2
  line L532 (-11.3563, 47.7798) -> (-10.8192, 45.7557)
  spline S393 degree 2 poles (-6.7247, 46.4249) (-7.1006, 46.3704) (-7.6878, 46.4861) (-7.9128, 46.6542) knots 0 0 0 1 2 2 2
  spline S394 degree 2 poles (-7.9128, 46.6542) (-8.169, 46.8425) (-8.4416, 47.4368) (-8.5075, 47.892) knots 0 0 0 1 2 2 2
  line L533 (-8.5075, 47.892) -> (-8.8921, 50.5474)
  line L534 (-8.8921, 50.5474) -> (-8.3265, 50.6293)
  line L535 (-8.3265, 50.6293) -> (-7.942, 47.9739)
  spline S395 degree 2 poles (-7.942, 47.9739) (-7.899, 47.6773) (-7.7652, 47.2882) (-7.6348, 47.1416) knots 0 0 0 1 2 2 2
  spline S396 degree 2 poles (-7.6348, 47.1416) (-7.4961, 46.9857) (-7.0775, 46.8667) (-6.7947, 46.9077) knots 0 0 0 1 2 2 2
  spline S397 degree 2 poles (-6.7947, 46.9077) (-6.5291, 46.9461) (-6.1408, 47.182) (-6.0519, 47.3709) knots 0 0 0 1 2 2 2
  spline S398 degree 2 poles (-6.0519, 47.3709) (-5.9685, 47.5484) (-5.95, 47.956) (-5.9915, 48.2422) knots 0 0 0 1 2 2 2
  line L536 (-5.9915, 48.2422) -> (-6.378, 50.9115)
  line L537 (-6.378, 50.9115) -> (-5.8125, 50.9934)
  line L538 (-5.8125, 50.9934) -> (-5.4279, 48.3379)
  spline S399 degree 2 poles (-5.4279, 48.3379) (-5.3635, 47.8931) (-5.4509, 47.2326) (-5.6471, 46.9823) knots 0 0 0 1 2 2 2
  spline S400 degree 2 poles (-5.6471, 46.9823) (-5.8216, 46.7528) (-6.3316, 46.4818) (-6.7247, 46.4249) knots 0 0 0 1 2 2 2
  line L539 (-1.8953, 46.9792) -> (-2.4377, 46.9425)
  line L540 (-2.4377, 46.9425) -> (-2.5618, 48.7782)
  spline S401 degree 2 poles (-2.5618, 48.7782) (-2.5769, 49.0007) (-2.6444, 49.3803) (-2.7148, 49.4908) knots 0 0 0 1 2 2 2
  spline S402 degree 2 poles (-2.7148, 49.4908) (-2.7891, 49.608) (-3.0335, 49.7102) (-3.2351, 49.6966) knots 0 0 0 1 2 2 2
  spline S403 degree 2 poles (-3.2351, 49.6966) (-3.4368, 49.683) (-3.8498, 49.4385) (-4.0432, 49.2508) knots 0 0 0 1 2 2 2
  line L541 (-4.0432, 49.2508) -> (-3.8805, 46.8449)
  line L542 (-3.8805, 46.8449) -> (-4.4228, 46.8082)
  line L543 (-4.4228, 46.8082) -> (-4.6406, 50.0276)
  line L544 (-4.6406, 50.0276) -> (-4.0982, 50.0643)
  line L545 (-4.0982, 50.0643) -> (-4.074, 49.7062)
  spline S404 degree 2 poles (-4.074, 49.7062) (-3.8454, 49.9417) (-3.3916, 50.2029) (-3.1274, 50.2208) knots 0 0 0 1 2 2 2
  spline S405 degree 2 poles (-3.1274, 50.2208) (-2.6546, 50.2528) (-2.0768, 49.6632) (-2.0366, 49.0687) knots 0 0 0 1 2 2 2
  line L546 (-2.0366, 49.0687) -> (-1.8953, 46.9792)
  line L547 (-0.5783, 46.9972) -> (-1.1219, 46.9874)
  line L548 (-1.1219, 46.9874) -> (-1.1802, 50.2136)
  line L549 (-1.1802, 50.2136) -> (-0.6367, 50.2234)
  line L550 (-0.6367, 50.2234) -> (-0.5783, 46.9972)
  line L551 (-0.6081, 50.7607) -> (-1.2248, 50.7495)
  line L552 (-1.2248, 50.7495) -> (-1.235, 51.3139)
  line L553 (-1.235, 51.3139) -> (-0.6183, 51.3251)
  line L554 (-0.6183, 51.3251) -> (-0.6081, 50.7607)
  line L555 (2.8408, 50.1674) -> (1.536, 46.9755)
  line L556 (1.536, 46.9755) -> (1.0484, 46.989)
  line L557 (1.0484, 46.989) -> (-0.0678, 50.2478)
  line L558 (-0.0678, 50.2478) -> (0.5209, 50.2315)
  line L559 (0.5209, 50.2315) -> (1.3336, 47.7236)
  line L560 (1.3336, 47.7236) -> (2.2765, 50.183)
  line L561 (2.2765, 50.183) -> (2.8408, 50.1674)
  spline S406 degree 2 poles (4.5495, 46.7064) (3.7792, 46.7775) (3.0123, 47.7196) (3.0859, 48.5176) knots 0 0 0 1 2 2 2
  spline S407 degree 2 poles (3.0859, 48.5176) (3.1583, 49.3018) (4.0664, 50.1559) (4.7292, 50.0947) knots 0 0 0 1 2 2 2
  spline S408 degree 2 poles (4.7292, 50.0947) (5.0276, 50.0672) (5.4731, 49.8511) (5.6261, 49.6515) knots 0 0 0 1 2 2 2
  spline S409 degree 2 poles (5.6261, 49.6515) (5.7827, 49.4516) (5.9176, 48.9037) (5.882, 48.5186) knots 0 0 0 1 2 2 2
  line L562 (5.882, 48.5186) -> (5.8548, 48.2237)
  line L563 (5.8548, 48.2237) -> (3.6306, 48.4289)
  spline S410 degree 2 poles (3.6306, 48.4289) (3.5791, 47.8702) (4.0865, 47.225) (4.5861, 47.1789) knots 0 0 0 1 2 2 2
  spline S411 degree 2 poles (4.5861, 47.1789) (4.7631, 47.1626) (5.114, 47.2107) (5.2585, 47.2603) knots 0 0 0 1 2 2 2
  spline S412 degree 2 poles (5.2585, 47.2603) (5.4107, 47.3163) (5.6231, 47.4192) (5.6942, 47.4686) knots 0 0 0 1 2 2 2
  line L564 (5.6942, 47.4686) -> (5.7254, 47.4657)
  line L565 (5.7254, 47.4657) -> (5.671, 46.8758)
  spline S413 degree 2 poles (5.671, 46.8758) (5.5738, 46.8463) (5.279, 46.7615) (5.1651, 46.7406) knots 0 0 0 1 2 2 2
  spline S414 degree 2 poles (5.1651, 46.7406) (5.0048, 46.7099) (4.7438, 46.6884) (4.5495, 46.7064) knots 0 0 0 1 2 2 2
  spline S415 degree 2 poles (5.3655, 48.6852) (5.3787, 48.9045) (5.318, 49.232) (5.2412, 49.3476) knots 0 0 0 1 2 2 2
  spline S416 degree 2 poles (5.2412, 49.3476) (5.1587, 49.4777) (4.8756, 49.6333) (4.657, 49.6535) knots 0 0 0 1 2 2 2
  spline S417 degree 2 poles (4.657, 49.6535) (4.4418, 49.6733) (4.1281, 49.5728) (3.9917, 49.4594) knots 0 0 0 1 2 2 2
  spline S418 degree 2 poles (3.9917, 49.4594) (3.8584, 49.3422) (3.705, 49.0449) (3.6687, 48.8418) knots 0 0 0 1 2 2 2
  line L566 (3.6687, 48.8418) -> (5.3655, 48.6852)
  line L567 (8.3374, 48.9507) -> (8.3098, 48.9548)
  spline S419 degree 2 poles (8.3098, 48.9548) (8.2503, 48.9813) (8.1169, 49.0082) (8.0239, 49.0221) knots 0 0 0 1 2 2 2
  spline S420 degree 2 poles (8.0239, 49.0221) (7.8067, 49.0544) (7.3511, 48.9285) (7.1304, 48.7711) knots 0 0 0 1 2 2 2
  line L568 (7.1304, 48.7711) -> (6.7933, 46.5066)
  line L569 (6.7933, 46.5066) -> (6.2556, 46.5867)
  line L570 (6.2556, 46.5867) -> (6.7308, 49.7783)
  line L571 (6.7308, 49.7783) -> (7.2684, 49.6982)
  line L572 (7.2684, 49.6982) -> (7.1976, 49.2226)
  spline S421 degree 2 poles (7.1976, 49.2226) (7.5296, 49.4409) (7.9991, 49.5894) (8.2059, 49.5586) knots 0 0 0 1 2 2 2
  spline S422 degree 2 poles (8.2059, 49.5586) (8.2886, 49.5463) (8.3703, 49.5271) (8.4205, 49.5091) knots 0 0 0 1 2 2 2
  line L573 (8.4205, 49.5091) -> (8.3374, 48.9507)
  spline S423 degree 2 poles (9.2015, 46.0123) (8.8838, 46.0762) (8.3682, 46.3577) (8.2063, 46.4898) knots 0 0 0 1 2 2 2
  line L574 (8.2063, 46.4898) -> (8.3266, 47.0876)
  line L575 (8.3266, 47.0876) -> (8.3539, 47.0821)
  spline S424 degree 2 poles (8.3539, 47.0821) (8.4113, 47.0137) (8.5696, 46.8468) (8.7089, 46.7441) knots 0 0 0 1 2 2 2
  spline S425 degree 2 poles (8.7089, 46.7441) (8.8291, 46.6524) (9.1378, 46.4908) (9.312, 46.4557) knots 0 0 0 1 2 2 2
  spline S426 degree 2 poles (9.312, 46.4557) (9.4384, 46.4303) (9.7405, 46.43) (9.8184, 46.464) knots 0 0 0 1 2 2 2
  spline S427 degree 2 poles (9.8184, 46.464) (9.9306, 46.509) (10.0489, 46.638) (10.0792, 46.7884) knots 0 0 0 1 2 2 2
  spline S428 degree 2 poles (10.0792, 46.7884) (10.117, 46.9762) (9.9512, 47.2122) (9.7012, 47.33) knots 0 0 0 1 2 2 2
  spline S429 degree 2 poles (9.7012, 47.33) (9.6035, 47.3746) (9.2893, 47.5089) (9.1568, 47.5746) knots 0 0 0 1 2 2 2
  spline S430 degree 2 poles (9.1568, 47.5746) (8.816, 47.7534) (8.576, 48.2566) (8.6385, 48.5675) knots 0 0 0 1 2 2 2
  spline S431 degree 2 poles (8.6385, 48.5675) (8.7251, 48.9979) (9.4787, 49.4044) (10.0116, 49.2971) knots 0 0 0 1 2 2 2
  spline S432 degree 2 poles (10.0116, 49.2971) (10.2747, 49.2442) (10.7815, 49.0072) (10.9426, 48.8717) knots 0 0 0 1 2 2 2
  line L576 (10.9426, 48.8717) -> (10.8278, 48.3012)
  line L577 (10.8278, 48.3012) -> (10.8005, 48.3067)
  spline S433 degree 2 poles (10.8005, 48.3067) (10.6285, 48.5119) (10.1676, 48.8001) (9.9113, 48.8517) knots 0 0 0 1 2 2 2
  spline S434 degree 2 poles (9.9113, 48.8517) (9.6483, 48.9046) (9.2415, 48.7554) (9.1968, 48.5334) knots 0 0 0 1 2 2 2
  spline S435 degree 2 poles (9.1968, 48.5334) (9.1563, 48.3318) (9.3323, 48.0938) (9.5591, 47.9842) knots 0 0 0 1 2 2 2
  spline S436 degree 2 poles (9.5591, 47.9842) (9.6691, 47.9301) (9.9505, 47.8095) (10.1035, 47.7396) knots 0 0 0 1 2 2 2
  spline S437 degree 2 poles (10.1035, 47.7396) (10.4341, 47.5807) (10.7076, 47.1027) (10.6368, 46.7508) knots 0 0 0 1 2 2 2
  spline S438 degree 2 poles (10.6368, 46.7508) (10.5955, 46.5459) (10.3621, 46.216) (10.1782, 46.1144) knots 0 0 0 1 2 2 2
  spline S439 degree 2 poles (10.1782, 46.1144) (9.9826, 46.008) (9.526, 45.947) (9.2015, 46.0123) knots 0 0 0 1 2 2 2
  line L578 (11.48, 45.5772) -> (10.9521, 45.707)
  line L579 (10.9521, 45.707) -> (11.7221, 48.8405)
  line L580 (11.7221, 48.8405) -> (12.25, 48.7108)
  line L581 (12.25, 48.7108) -> (11.48, 45.5772)
  line L582 (12.4153, 49.2227) -> (11.8163, 49.3699)
  line L583 (11.8163, 49.3699) -> (11.951, 49.9181)
  line L584 (11.951, 49.9181) -> (12.55, 49.7709)
  line L585 (12.55, 49.7709) -> (12.4153, 49.2227)
  spline S440 degree 2 poles (13.1742, 45.0521) (12.7485, 45.1729) (12.407, 45.7949) (12.5563, 46.3213) knots 0 0 0 1 2 2 2
  line L586 (12.5563, 46.3213) -> (13.0441, 48.041)
  line L587 (13.0441, 48.041) -> (12.6921, 48.1409)
  line L588 (12.6921, 48.1409) -> (12.8148, 48.5733)
  line L589 (12.8148, 48.5733) -> (13.1668, 48.4735)
  line L590 (13.1668, 48.4735) -> (13.4197, 49.3652)
  line L591 (13.4197, 49.3652) -> (13.9427, 49.2168)
  line L592 (13.9427, 49.2168) -> (13.6898, 48.3251)
  line L593 (13.6898, 48.3251) -> (14.6519, 48.0522)
  line L594 (14.6519, 48.0522) -> (14.5292, 47.6197)
  line L595 (14.5292, 47.6197) -> (13.5671, 47.8927)
  line L596 (13.5671, 47.8927) -> (13.1477, 46.4143)
  spline S441 degree 2 poles (13.1477, 46.4143) (13.0812, 46.1796) (13.0247, 45.9167) (13.0503, 45.7899) knots 0 0 0 1 2 2 2
  spline S442 degree 2 poles (13.0503, 45.7899) (13.0697, 45.6794) (13.2533, 45.5223) (13.4343, 45.4709) knots 0 0 0 1 2 2 2
  spline S443 degree 2 poles (13.4343, 45.4709) (13.5617, 45.4348) (13.8216, 45.4444) (13.8819, 45.4526) knots 0 0 0 1 2 2 2
  line L597 (13.8819, 45.4526) -> (13.9121, 45.4441)
  line L598 (13.9121, 45.4441) -> (13.7789, 44.9747)
  spline S444 degree 2 poles (13.7789, 44.9747) (13.62, 44.9764) (13.305, 45.015) (13.1742, 45.0521) knots 0 0 0 1 2 2 2
  spline S445 degree 2 poles (15.9665, 44.5724) (15.8881, 44.5477) (15.6206, 44.4553) (15.5047, 44.4398) knots 0 0 0 1 2 2 2
  spline S446 degree 2 poles (15.5047, 44.4398) (15.3447, 44.4136) (15.0649, 44.4249) (14.8342, 44.504) knots 0 0 0 1 2 2 2
  spline S447 degree 2 poles (14.8342, 44.504) (14.6463, 44.5685) (14.3554, 44.8266) (14.271, 44.9993) knots 0 0 0 1 2 2 2
  spline S448 degree 2 poles (14.271, 44.9993) (14.192, 45.1664) (14.1703, 45.5864) (14.2404, 45.7908) knots 0 0 0 1 2 2 2
  spline S449 degree 2 poles (14.2404, 45.7908) (14.349, 46.1072) (14.7697, 46.4639) (15.1039, 46.4929) knots 0 0 0 1 2 2 2
  spline S450 degree 2 poles (15.1039, 46.4929) (15.4017, 46.5234) (16.131, 46.3727) (16.5443, 46.2567) knots 0 0 0 1 2 2 2
  line L599 (16.5443, 46.2567) -> (16.5782, 46.3555)
  spline S451 degree 2 poles (16.5782, 46.3555) (16.6393, 46.5335) (16.6063, 46.7917) (16.5289, 46.8882) knots 0 0 0 1 2 2 2
  spline S452 degree 2 poles (16.5289, 46.8882) (16.4515, 46.9848) (16.1816, 47.1216) (16.03, 47.1736) knots 0 0 0 1 2 2 2
  spline S453 degree 2 poles (16.03, 47.1736) (15.852, 47.2346) (15.3346, 47.2942) (15.0589, 47.2746) knots 0 0 0 1 2 2 2
  line L600 (15.0589, 47.2746) -> (15.0292, 47.2848)
  line L601 (15.0292, 47.2848) -> (15.209, 47.8088)
  spline S454 degree 2 poles (15.209, 47.8088) (15.3643, 47.7998) (15.9289, 47.7166) (16.1893, 47.6273) knots 0 0 0 1 2 2 2
  spline S455 degree 2 poles (16.1893, 47.6273) (16.5057, 47.5187) (16.9036, 47.2717) (17.0309, 47.0844) knots 0 0 0 1 2 2 2
  spline S456 degree 2 poles (17.0309, 47.0844) (17.156, 46.9015) (17.184, 46.4461) (17.0856, 46.1594) knots 0 0 0 1 2 2 2
  line L602 (17.0856, 46.1594) -> (16.3699, 44.073)
  line L603 (16.3699, 44.073) -> (15.8557, 44.2494)
  line L604 (15.8557, 44.2494) -> (15.9665, 44.5724)
  line L605 (16.1135, 45.0009) -> (16.4041, 45.8479)
  spline S457 degree 2 poles (16.4041, 45.8479) (16.2139, 45.8948) (15.6376, 46.0298) (15.4448, 46.037) knots 0 0 0 1 2 2 2
  spline S458 degree 2 poles (15.4448, 46.037) (15.219, 46.0445) (14.8627, 45.8757) (14.7835, 45.645) knots 0 0 0 1 2 2 2
  spline S459 degree 2 poles (14.7835, 45.645) (14.6931, 45.3813) (14.8981, 45.0126) (15.1816, 44.9153) knots 0 0 0 1 2 2 2
  spline S460 degree 2 poles (15.1816, 44.9153) (15.4222, 44.8328) (15.889, 44.9047) (16.1135, 45.0009) knots 0 0 0 1 2 2 2
  line L606 (17.2823, 47.7423) -> (16.7319, 47.9311)
  line L607 (16.7319, 47.9311) -> (16.9151, 48.4651)
  line L608 (16.9151, 48.4651) -> (17.4655, 48.2762)
  line L609 (17.4655, 48.2762) -> (17.2823, 47.7423)
  line L610 (16.1551, 48.129) -> (15.6047, 48.3178)
  line L611 (15.6047, 48.3178) -> (15.7878, 48.8518)
  line L612 (15.7878, 48.8518) -> (16.3383, 48.6629)
  line L613 (16.3383, 48.6629) -> (16.1551, 48.129)
  spline S461 degree 2 poles (17.9598, 43.367) (17.5495, 43.533) (17.2772, 44.1883) (17.4824, 44.6955) knots 0 0 0 1 2 2 2
  line L614 (17.4824, 44.6955) -> (18.153, 46.3525)
  line L615 (18.153, 46.3525) -> (17.8138, 46.4898)
  line L616 (17.8138, 46.4898) -> (17.9825, 46.9065)
  line L617 (17.9825, 46.9065) -> (18.3216, 46.7692)
  line L618 (18.3216, 46.7692) -> (18.6693, 47.6284)
  line L619 (18.6693, 47.6284) -> (19.1732, 47.4245)
  line L620 (19.1732, 47.4245) -> (18.8255, 46.5653)
  line L621 (18.8255, 46.5653) -> (19.7526, 46.1901)
  line L622 (19.7526, 46.1901) -> (19.5839, 45.7734)
  line L623 (19.5839, 45.7734) -> (18.6569, 46.1486)
  line L624 (18.6569, 46.1486) -> (18.0804, 44.7241)
  spline S462 degree 2 poles (18.0804, 44.7241) (17.9889, 44.498) (17.9044, 44.2427) (17.9162, 44.1139) knots 0 0 0 1 2 2 2
  spline S463 degree 2 poles (17.9162, 44.1139) (17.9235, 44.002) (18.0891, 43.8259) (18.2635, 43.7553) knots 0 0 0 1 2 2 2
  spline S464 degree 2 poles (18.2635, 43.7553) (18.3863, 43.7057) (18.6457, 43.6872) (18.7065, 43.6888) knots 0 0 0 1 2 2 2
  line L625 (18.7065, 43.6888) -> (18.7356, 43.6771)
  line L626 (18.7356, 43.6771) -> (18.5526, 43.2249)
  spline S465 degree 2 poles (18.5526, 43.2249) (18.3948, 43.2436) (18.0857, 43.316) (17.9598, 43.367) knots 0 0 0 1 2 2 2
  spline S466 degree 2 poles (21.6532, 41.6286) (21.239, 41.8442) (20.748, 42.3197) (20.5558, 42.5769) knots 0 0 0 1 2 2 2
  line L627 (20.5558, 42.5769) -> (20.8872, 43.2136)
  line L628 (20.8872, 43.2136) -> (20.9243, 43.1943)
  spline S467 degree 2 poles (20.9243, 43.1943) (21.0524, 42.8291) (21.5509, 42.2397) (21.8445, 42.0868) knots 0 0 0 1 2 2 2
  spline S468 degree 2 poles (21.8445, 42.0868) (22.2649, 41.868) (22.8764, 41.9937) (23.026, 42.2811) knots 0 0 0 1 2 2 2
  spline S469 degree 2 poles (23.026, 42.2811) (23.145, 42.5099) (23.0674, 42.9117) (22.8602, 43.1099) knots 0 0 0 1 2 2 2
  spline S470 degree 2 poles (22.8602, 43.1099) (22.7098, 43.251) (22.4515, 43.4719) (22.261, 43.6417) knots 0 0 0 1 2 2 2
  spline S471 degree 2 poles (22.261, 43.6417) (22.0905, 43.7972) (21.8604, 44.1174) (21.8058, 44.3068) knots 0 0 0 1 2 2 2
  spline S472 degree 2 poles (21.8058, 44.3068) (21.7543, 44.4947) (21.8015, 44.9023) (21.9173, 45.1248) knots 0 0 0 1 2 2 2
  spline S473 degree 2 poles (21.9173, 45.1248) (22.1586, 45.5885) (23.2085, 45.8395) (23.768, 45.5483) knots 0 0 0 1 2 2 2
  spline S474 degree 2 poles (23.768, 45.5483) (24.0894, 45.381) (24.5922, 44.9582) (24.7737, 44.7106) knots 0 0 0 1 2 2 2
  line L629 (24.7737, 44.7106) -> (24.4583, 44.1048)
  line L630 (24.4583, 44.1048) -> (24.4212, 44.1241)
  spline S475 degree 2 poles (24.4212, 44.1241) (24.3257, 44.3859) (23.8857, 44.9292) (23.5735, 45.0917) knots 0 0 0 1 2 2 2
  spline S476 degree 2 poles (23.5735, 45.0917) (23.2211, 45.2751) (22.6132, 45.1712) (22.4732, 44.9023) knots 0 0 0 1 2 2 2
  spline S477 degree 2 poles (22.4732, 44.9023) (22.3477, 44.6612) (22.4547, 44.2402) (22.662, 44.0498) knots 0 0 0 1 2 2 2
  spline S478 degree 2 poles (22.662, 44.0498) (22.8002, 43.9229) (23.209, 43.5687) (23.3394, 43.4419) knots 0 0 0 1 2 2 2
  spline S479 degree 2 poles (23.3394, 43.4419) (23.6692, 43.117) (23.7814, 42.4419) (23.5964, 42.0864) knots 0 0 0 1 2 2 2
  spline S480 degree 2 poles (23.5964, 42.0864) (23.4789, 41.8608) (23.0713, 41.5229) (22.8287, 41.4567) knots 0 0 0 1 2 2 2
  spline S481 degree 2 poles (22.8287, 41.4567) (22.5594, 41.3848) (22.0025, 41.4468) (21.6532, 41.6286) knots 0 0 0 1 2 2 2
  spline S482 degree 2 poles (25.2071, 40.0777) (25.1252, 40.0706) (24.8441, 40.038) (24.7276, 40.0479) knots 0 0 0 1 2 2 2
  spline S483 degree 2 poles (24.7276, 40.0479) (24.5657, 40.0569) (24.295, 40.1282) (24.0867, 40.2553) knots 0 0 0 1 2 2 2
  spline S484 degree 2 poles (24.0867, 40.2553) (23.9172, 40.3588) (23.6889, 40.6736) (23.6437, 40.8604) knots 0 0 0 1 2 2 2
  spline S485 degree 2 poles (23.6437, 40.8604) (23.6026, 41.0406) (23.672, 41.4554) (23.7846, 41.6399) knots 0 0 0 1 2 2 2
  spline S486 degree 2 poles (23.7846, 41.6399) (23.9588, 41.9254) (24.4467, 42.1829) (24.7792, 42.1392) knots 0 0 0 1 2 2 2
  spline S487 degree 2 poles (24.7792, 42.1392) (25.0766, 42.1047) (25.7562, 41.8001) (26.1347, 41.5977) knots 0 0 0 1 2 2 2
  line L631 (26.1347, 41.5977) -> (26.1892, 41.6869)
  spline S488 degree 2 poles (26.1892, 41.6869) (26.2872, 41.8476) (26.3107, 42.1067) (26.2559, 42.2177) knots 0 0 0 1 2 2 2
  spline S489 degree 2 poles (26.2559, 42.2177) (26.2012, 42.3287) (25.9671, 42.5205) (25.8303, 42.604) knots 0 0 0 1 2 2 2
  spline S490 degree 2 poles (25.8303, 42.604) (25.6697, 42.702) (25.1773, 42.8718) (24.9039, 42.9122) knots 0 0 0 1 2 2 2
  line L632 (24.9039, 42.9122) -> (24.8772, 42.9285)
  line L633 (24.8772, 42.9285) -> (25.1658, 43.4014)
  spline S491 degree 2 poles (25.1658, 43.4014) (25.3155, 43.3591) (25.8488, 43.1561) (26.0838, 43.0126) knots 0 0 0 1 2 2 2
  spline S492 degree 2 poles (26.0838, 43.0126) (26.3693, 42.8384) (26.7045, 42.5114) (26.7884, 42.301) knots 0 0 0 1 2 2 2
  spline S493 degree 2 poles (26.7884, 42.301) (26.8711, 42.0954) (26.8002, 41.6447) (26.6423, 41.3859) knots 0 0 0 1 2 2 2
  line L634 (26.6423, 41.3859) -> (25.4933, 39.5031)
  line L635 (25.4933, 39.5031) -> (25.0293, 39.7862)
  line L636 (25.0293, 39.7862) -> (25.2071, 40.0777)
  line L637 (25.4431, 40.4644) -> (25.9096, 41.2289)
  spline S494 degree 2 poles (25.9096, 41.2289) (25.734, 41.3156) (25.2004, 41.5718) (25.0138, 41.6205) knots 0 0 0 1 2 2 2
  spline S495 degree 2 poles (25.0138, 41.6205) (24.7948, 41.6765) (24.4105, 41.5885) (24.2834, 41.3803) knots 0 0 0 1 2 2 2
  spline S496 degree 2 poles (24.2834, 41.3803) (24.1382, 41.1424) (24.2589, 40.7381) (24.5147, 40.582) knots 0 0 0 1 2 2 2
  spline S497 degree 2 poles (24.5147, 40.582) (24.7318, 40.4495) (25.2031, 40.419) (25.4431, 40.4644) knots 0 0 0 1 2 2 2
  line L638 (26.5819, 38.7618) -> (26.1318, 39.0666)
  line L639 (26.1318, 39.0666) -> (28.6507, 42.7855)
  line L640 (28.6507, 42.7855) -> (29.1008, 42.4807)
  line L641 (29.1008, 42.4807) -> (26.5819, 38.7618)
  line L642 (28.943, 37.0505) -> (27.0391, 38.4611)
  line L643 (27.0391, 38.4611) -> (27.2797, 38.7859)
  line L644 (27.2797, 38.7859) -> (30.0496, 39.6914)
  line L645 (30.0496, 39.6914) -> (28.7505, 40.6539)
  line L646 (28.7505, 40.6539) -> (29.016, 41.0123)